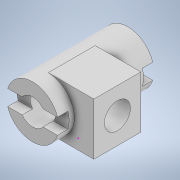
# Autodesk Inventor part: Część2
Saved by Autodesk Inventor 2021 (Build 250183000, 183)
## iProperties
Created: 2024-04-13
Part Number: Część2
Material: Ogólny
Document SubType Name: Modeling
Designer: Dawidek
Density: 1 g/cm^3
Appearance: Domyślna
Author: Dawidek
Autodesk Inventor part; units mm, degrees
ref_plane "YZ Plane" through (0, 0, 0) normal (1, 0, 0) x (0, 1, 0)
sketch "Szkic1" plane through (0, 0, 0) normal (0, 0, 1) x (1, 0, 0)
  circle A0 centre (0, 0) radius 20
  circle A1 centre (0, 0) radius 10
  dimension "d0" = 40
  dimension "d1" = 20
  constraints: 2 centre point, 2 coincident
  measures "d0" diameter of A0
  measures "d1" diameter of A1
extrude "Wyciągnięcie proste1" add sketch "Szkic1" against normal blind 73
sketch "Szkic2" plane through (0, 0, 0) normal (0, 0, 1) x (1, 0, 0)
  line L0 (0, 0) -> (0, 6)
  line L1 (0, 6) -> (24.4781, 6)
  line L2 (24.4781, 6) -> (24.4781, -6)
  line L3 (24.4781, -6) -> (-24.6977, -6)
  line L4 (-24.6977, -6) -> (-24.6977, 6)
  line L5 (-24.6977, 6) -> (0, 6)
  dimension "d4" = 6
  dimension "d5" = 12
  constraints: 12 end point, 5 perpendicular, 1 point on line, 1 vertical
  measures "d4" distance of L0.start L0.end
  measures "d5" distance of L1.end L2.end
extrude "Wyciągnięcie proste2" cut sketch "Szkic2" against normal blind 8
sketch "Szkic3" plane through (0, 0, -73) normal (0, 0, -1) x (-1, 0, 0)
  line L0 (0, 0) -> (23.7964, 0)
  line L1 (0, 0) -> (26.8721, 0)
  line L2 (26.8721, 0) -> (26.8721, 6)
  line L3 (26.8721, 6) -> (-29.6241, 6)
  line L4 (-29.6241, 6) -> (-29.6241, -6)
  line L5 (-29.6241, -6) -> (26.8721, -6)
  line L6 (26.8721, -6) -> (26.8721, 0)
  dimension "d8" = 6
  dimension "d9" = 12
  constraints: 14 end point, 4 perpendicular, 1 horizontal, 1 point on line, 1 vertical
  measures "d8" distance of L1.end L2.end
  measures "d9" distance of L3.end L4.end
extrude "Wyciągnięcie proste3" cut sketch "Szkic3" against normal blind 8
ref_plane "Płaszczyzna konstrukcyjna1" through (35, -6, 0) normal (1, 0, 0) x (0, 0, -1)
sketch "Szkic5" plane through (35, -6, 0) normal (1, 0, 0) x (0, 0, -1)
  point P0 (0, 6)
ref_plane "Płaszczyzna konstrukcyjna2" through (35, -6, 0) normal (1, 0, 0) x (0, 0, -1)
sketch "Szkic6" plane through (35, -6, 0) normal (1, 0, 0) x (0, 0, -1)
  line L0 (12, 0) -> (12, 2) projected
  line L1 (12, 2) -> (12, 26)
  line L2 (0, 26) -> (73, 26) projected
  line L3 (12, 26) -> (48, 26)
  line L4 (48, 26) -> (48, -14)
  line L5 (0, -14) -> (73, -14) projected
  line L6 (12, -14) -> (12, 2)
  line L7 (12, 0) -> (0, 0) projected
  point P0 (0, 6)
  dimension "d16" = 36
  constraints: 8 end point, 4 point on line, 2 perpendicular, 1 vertical
  measures "d16" distance of L1.end L3.end
extrude "Wyciągnięcie proste5" add sketch "Szkic6" against normal blind 35
sketch "Szkic7" plane through (0, 0, -12) normal (0, 0, 1) x (1, 0, 0)
  circle A0 centre (0, 0) radius 10
  dimension "d19" = 20
  constraints: 1 centre point, 1 coincident
  measures "d19" diameter of A0
extrude "Wyciągnięcie proste6" cut sketch "Szkic7" against normal blind 65
sketch "Szkic8" plane through (35, -6, 0) normal (1, 0, 0) x (0, 0, -1)
  line L0 (12, 26) -> (12, -14) projected
  circle A0 centre (30, 6) radius 10
  point P0 (0, 6)
  dimension "d24" = 20
  constraints: 1 centre point
  measures "d24" diameter of A0
extrude "Wyciągnięcie proste7" cut sketch "Szkic8" against normal blind 35
